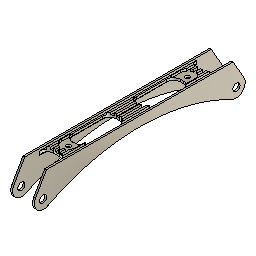
Sample Wall 270mm (Autodesk Fusion 360 archive; units mm, degrees)
design "Core-Large CDK"
Autodesk Fusion 360 part; units mm, degrees
sketch "Sketch1" plane through (0, 0, 0) normal (1, 0, 0) x (0, 1, 0)
  circle A0 centre (-135, -8) radius 5.05
  circle A1 centre (135, -8) radius 5.05
  arc A2 (128.3341, -19.5451) -> (-128.3341, -19.5451) centre (0, -267.4784) ccw
  line L0 (0, 25) -> (0, 11.7) construction
  arc A3 (-145.5683, -1.5) -> (-128.3341, -19.5451) centre (-134.31, -8) ccw
  line L1 (-20, 11.7) -> (20, 11.7) construction
  arc A4 (128.3341, -19.5451) -> (145.5683, -1.5) centre (134.31, -8) ccw
  line L2 (-135, -8) -> (135, -8) construction
  line L3 (-130.2685, 25) -> (130.2685, 25)
  line L4 (-132.0006, 22) -> (132.0006, 22)
  line L5 (-145.5683, -1.5) -> (-130.2685, 25)
  line L6 (145.5683, -1.5) -> (130.2685, 25)
  dimension "d3" = 10.1
  dimension "d4" = 135
  dimension "d5" = 10.1
  dimension "d6" = 135
  dimension "d146" = 13.3
  dimension "d154" = 13
  dimension "d155" = 25
  dimension "d156" = 33
  dimension "d157" = 120
  dimension "d158" = 13
  dimension "d159" = 120
  dimension "d160" = 0.69
  dimension "d161" = 0.69
  dimension "d162" = 3
  constraint horizontal L1
  constraint midpoint L0.end L1
  constraint tangent A2 A4
  constraint tangent A2 A3
  constraint coincident A0.centre L2.start
  constraint coincident A1.centre L2.end
  constraint horizontal L2
  constraint coincident L0.start L3
  constraint coincident L4.start L5
  constraint tangent A3 L5
  constraint coincident L4.end L6
  constraint tangent A4 L6
  constraint coincident A3.centre L2
  constraint coincident A4.centre L2
  constraint tangent A2 L1
  constraint horizontal L4
  measures "d3" diameter of A0
  measures "d4" horizontal distance of origin A0.centre
  measures "d5" diameter of A1
  measures "d6" horizontal distance of origin A1.centre
  measures "d146" distance of L0.start L0.end
  measures "d154" radius of A3
  measures "d155" distance of origin L0.start
  measures "d156" distance of L2 L3
  measures "d157" angle of L3 L5
  measures "d158" radius of A4
  measures "d159" angle of L3 L6
  measures "d160" distance of A3.centre A0.centre
  measures "d161" distance of A1.centre A4.centre
  measures "d162" distance of L3 L4
extrude "Extrude1" add sketch "Sketch1" along normal mid plane 33 makes body 1
sketch "Sketch3" plane through (0, 0, 0) normal (0, 1, 0) x (1, 0, 0)
  line L0 (-11.5, -19) -> (11.5, -19)
  line L1 (14, -16.5) -> (14, 23)
  line L2 (14, 23) -> (-14, 23)
  line L3 (-14, 23) -> (-14, -16.5)
  line L4 (-14, -19) -> (14, 23) construction
  line L5 (14, -19) -> (-14, 23) construction
  line L6 (-16.5, -22) -> (16.5, -22)
  line L7 (-11, -22) -> (-14, -22)
  line L8 (-14, -22) -> (-14, -25)
  line L9 (-14, -25) -> (-11, -25)
  line L10 (-11, -25) -> (-11, -22)
  line L11 (-11, -22) -> (-14, -25) construction
  line L12 (-14, -22) -> (-11, -25) construction
  line L13 (-16.5, 1.4544) -> (-16.5, -22)
  line L14 (14, -22) -> (11, -22)
  line L15 (11, -22) -> (11, -25)
  line L16 (11, -25) -> (14, -25)
  line L17 (14, -25) -> (14, -22)
  line L18 (14, -22) -> (11, -25) construction
  line L19 (11, -22) -> (14, -25) construction
  line L20 (16.5, -22) -> (16.5, 1.4544)
  arc A0 (-14, -16.5) -> (-11.5, -19) centre (-11.5, -16.5) ccw
  arc A1 (11.5, -19) -> (14, -16.5) centre (11.5, -16.5) ccw
  line L21 (5, -22) -> (8, -22)
  line L22 (8, -22) -> (8, -25)
  line L23 (8, -25) -> (5, -25)
  line L24 (5, -25) -> (5, -22)
  line L25 (5, -22) -> (8, -25) construction
  line L26 (8, -22) -> (5, -25) construction
  line L27 (-8, -22) -> (-5, -22)
  line L28 (-5, -22) -> (-5, -25)
  line L29 (-5, -25) -> (-8, -25)
  line L30 (-8, -25) -> (-8, -22)
  line L31 (-8, -22) -> (-5, -25) construction
  line L32 (-5, -22) -> (-8, -25) construction
  line L33 (-2, -22) -> (2, -22)
  line L34 (2, -22) -> (2, -25)
  line L35 (2, -25) -> (-2, -25)
  line L36 (-2, -25) -> (-2, -22)
  line L37 (-2, -22) -> (2, -25) construction
  line L38 (2, -22) -> (-2, -25) construction
  line L39 (-16.5, -25) -> (16.5, -25)
  point P0 (0, 2)
  point P1 (-12.5, -23.5)
  point P2 (12.5, -23.5)
  point P3 (0, -20.5)
  point P4 (6.5, -23.5)
  point P5 (-6.5, -23.5)
  point P6 (0, -23.5)
  dimension "d22" = 28
  dimension "d24" = 42
  dimension "d79" = 3
  dimension "d80" = 3
  dimension "d81" = 2.5
  dimension "d82" = 3
  dimension "d83" = 3
  dimension "d84" = 2.5
  dimension "d101" = 2.5
  dimension "d102" = 2.5
  dimension "d103" = 3
  dimension "d104" = 3
  dimension "d105" = 3
  dimension "d106" = 3
  dimension "d107" = 3
  dimension "d108" = 3
  dimension "d109" = 4
  dimension "d110" = 3
  dimension "d147" = 6
  constraint horizontal L0
  constraint perpendicular L0 L1
  constraint parallel L0 L2
  constraint parallel L1 L3
  constraint coincident L4 P0
  constraint coincident L5 P0
  constraint horizontal L7
  constraint perpendicular L7 L8
  constraint parallel L7 L9
  constraint parallel L8 L10
  constraint coincident L11 P1
  constraint coincident L12 P1
  constraint horizontal L14
  constraint perpendicular L14 L15
  constraint parallel L14 L16
  constraint parallel L15 L17
  constraint coincident L18 P2
  constraint coincident L19 P2
  constraint vertical origin P3
  constraint coincident L4.start L0
  constraint coincident L4.start L3
  constraint tangent L0 A0
  constraint tangent L3 A0
  constraint coincident L5.start L0
  constraint coincident L5.start L1
  constraint tangent L0 A1
  constraint tangent L1 A1
  constraint vertical origin P0
  constraint horizontal L21
  constraint perpendicular L21 L22
  constraint parallel L21 L23
  constraint parallel L22 L24
  constraint coincident L25 P4
  constraint coincident L26 P4
  constraint horizontal L27
  constraint perpendicular L27 L28
  constraint parallel L27 L29
  constraint parallel L28 L30
  constraint coincident L31 P5
  constraint coincident L32 P5
  constraint horizontal L33
  constraint perpendicular L33 L34
  constraint parallel L33 L35
  constraint parallel L34 L36
  constraint coincident L37 P6
  constraint coincident L38 P6
  constraint vertical P0 P6
  constraint horizontal L15.end L39.end
  constraint horizontal L34.end L39.end
  constraint horizontal L28.end L39.end
  measures "d22" distance of L1.end L2.end
  measures "d24" distance of L0 L2
  measures "d79" distance of L8.end L9.end
  measures "d80" distance of L7.end L8.end
  measures "d81" distance of L8 L13
  measures "d82" distance of L15.end L16.end
  measures "d83" distance of L14.end L15.end
  measures "d84" distance of L17 L20
  measures "d101" radius of A0
  measures "d102" radius of A1
  measures "d103" distance of L22.end L23.end
  measures "d104" distance of L21.end L22.end
  measures "d105" distance of L15 L22
  measures "d106" distance of L28.end L29.end
  measures "d107" distance of L27.end L28.end
  measures "d108" distance of L10 L30
  measures "d109" distance of L34.end L35.end
  measures "d110" distance of L33.end L34.end
  measures "d147" distance of L0 L39
extrude "Extrude2" cut sketch "Sketch3" along normal mid plane 360 contours L0 L1 L2 L3 A0 A1 | L6 L7 L8 L9 L10 L39 | L6 L27 L28 L29 L30 L39 | L6 L33 L34 L35 L36 L39 | L6 L21 L22 L23 L24 L39 | L6 L14 L15 L16 L17 L39 bodies 1
sketch "Sketch4" plane through (0, 0, 25) normal (0, 0, 1) x (-1, 0, 0)
  line L0 (-14, 122) -> (-16.5, 122)
  line L1 (-16.5, 122) -> (-16.5, -122)
  line L2 (-16.5, -122) -> (-14, -122)
  line L3 (16.5, -122) -> (16.5, 122)
  line L4 (0, 0) -> (0, -83.5) construction
  line L5 (0, 0) -> (0, 83.5) construction
  circle A0 centre (0, -83.5) radius 10.1
  circle A1 centre (0, -83.5) radius 3.1
  circle A2 centre (0, 83.5) radius 10.1
  circle A3 centre (0, 83.5) radius 3.1
  line L6 (-14, -122) -> (-14, 122)
  line L7 (14, 122) -> (14, -122)
  line L8 (14, -122) -> (16.5, -122)
  line L9 (16.5, 122) -> (14, 122)
  line L10 (-14, 25) -> (14, 25)
  line L11 (14, 25) -> (14, -25)
  line L12 (14, -25) -> (-14, -25)
  line L13 (-14, -25) -> (-14, 25)
  line L14 (-14, 25) -> (14, -25) construction
  line L15 (14, 25) -> (-14, -25) construction
  line L16 (-10.1, -63.49) -> (10.1, -63.49)
  line L17 (10.1, -63.49) -> (10.1, -83.5)
  line L18 (10.1, -83.5) -> (-10.1, -83.5)
  line L19 (-10.1, -83.5) -> (-10.1, -63.49)
  line L20 (-10.1, -63.49) -> (10.1, -83.5) construction
  line L21 (10.1, -63.49) -> (-10.1, -83.5) construction
  line L22 (-10.1, 83.5) -> (10.1, 83.5)
  line L23 (10.1, 83.5) -> (10.1, 63.48)
  line L24 (10.1, 63.48) -> (-10.1, 63.48)
  line L25 (-10.1, 63.48) -> (-10.1, 83.5)
  line L26 (-10.1, 83.5) -> (10.1, 63.48) construction
  line L27 (10.1, 83.5) -> (-10.1, 63.48) construction
  line L28 (-2, -132.0006) -> (2, -132.0006)
  line L29 (2, -132.0006) -> (2, 132.0006)
  line L30 (2, 132.0006) -> (-2, 132.0006)
  line L31 (-2, 132.0006) -> (-2, -132.0006)
  line L32 (-14, -130.2685) -> (-14, 130.2685)
  line L33 (-14, 130.2685) -> (-16.5, 130.2685)
  line L34 (-16.5, 130.2685) -> (-16.5, -130.2685)
  line L35 (-16.5, -130.2685) -> (-14, -130.2685)
  point P0 (0, -73.495)
  point P1 (0, 73.49)
  dimension "d28" = 83.5
  dimension "d29" = 83.5
  dimension "d30" = 20.2
  dimension "d31" = 6.2
  dimension "d32" = 20.2
  dimension "d33" = 6.2
  dimension "d97" = 28
  dimension "d98" = 50
  dimension "d125" = 20.01
  dimension "d126" = 20.2
  dimension "d127" = 20.2
  dimension "d128" = 20.02
  constraint coincident L4.start L5.start
  constraint vertical L4
  constraint parallel L4 L5
  constraint coincident L4.end A0.centre
  constraint concentric A0 A1
  constraint coincident L5.end A2.centre
  constraint concentric A2 A3
  constraint horizontal L10
  constraint perpendicular L10 L11
  constraint parallel L10 L12
  constraint parallel L11 L13
  constraint coincident L14 L4.start
  constraint coincident L15 L4.start
  constraint horizontal L16
  constraint perpendicular L16 L17
  constraint parallel L16 L18
  constraint parallel L17 L19
  constraint coincident L20 P0
  constraint coincident L21 P0
  constraint coincident L4 P0
  constraint horizontal L4.end L17.end
  constraint horizontal L22
  constraint perpendicular L22 L23
  constraint parallel L22 L24
  constraint parallel L23 L25
  constraint coincident L26 P1
  constraint coincident L27 P1
  constraint coincident L5 P1
  constraint horizontal L5.end L22.end
  measures "d28" distance of L4.start L4.end
  measures "d29" distance of L4.start L5.end
  measures "d30" diameter of A0
  measures "d31" diameter of A1
  measures "d32" diameter of A2
  measures "d33" diameter of A3
  measures "d97" distance of L11.end L12.end
  measures "d98" distance of L10.end L11.end
  measures "d125" distance of L16.end L17.end
  measures "d126" distance of L17 L19
  measures "d127" distance of L23.end L24.end
  measures "d128" distance of L22.end L23.end
extrude "Extrude3" cut sketch "Sketch4" against normal blind 100 contours A3 L22 L29 L31 | A3 L22 L31 | A1 L18 L31 | A1 L18 L29 L31 | A3 L22 L29 | A3 L22 L31 | A3 L22 L29 L31 | A1 L18 L29 | A1 L18 L31 | A1 L18 L29 L31 | A3 L22 L29 | A1 L18 L29 bodies 1
sketch "Sketch5" plane through (0, 0, 19) normal (0, 0, -1) x (1, 0, 0)
  circle A0 centre (0, -83.5) radius 3.1
  circle A1 centre (0, 83.5) radius 3.1
  circle A2 centre (0, -83.5) radius 13.1
  circle A3 centre (0, 83.5) radius 13.1
  line L0 (-11.5, 133.7326) -> (-11.5, -133.7326)
  line L1 (11.5, -133.7326) -> (11.5, 133.7326)
  line L2 (11.5, 133.7326) -> (-11.5, 133.7326)
  line L3 (-11.5, -133.7326) -> (11.5, -133.7326)
  dimension "d36" = 26.2
  dimension "d37" = 26.2
  constraint concentric A0 A2
  constraint concentric A1 A3
  measures "d36" diameter of A2
  measures "d37" diameter of A3
extrude "Extrude5" cut sketch "Sketch4" against normal blind 3 contours A2 L24 L29 L31 | A2 L24 L25 L31 | A0 L16 L19 L31 | A0 L16 L29 L31 | A2 L23 L24 L29 | A2 A3 L29 L31 | A2 A3 L22 L31 | A0 L16 L17 L29 | A0 A1 L18 L31 | A0 A1 L29 L31 | A2 A3 L22 L29 | A2 A3 L22 L31 | A0 A1 L18 L29 | A0 A1 L18 L31 | A2 A3 L22 L29 | A2 A3 L29 L31 | A0 A1 L18 L29 | A0 A1 L29 L31 bodies 1
sketch "Sketch6" plane through (0, 0, 25) normal (0, 0, 1) x (-1, 0, 0)
  line L0 (-14, 122) -> (-16.5, 122)
  line L1 (-16.5, 122) -> (-16.5, -122)
  line L2 (-16.5, -122) -> (-14, -122)
  line L3 (16.5, -122) -> (16.5, 122)
  line L4 (14, 149.5) -> (-14, 149.5)
  line L5 (-14, 149.5) -> (-14, 109.6)
  line L6 (-3.9, 99.5) -> (3.9, 99.5)
  line L7 (14, 109.6) -> (14, 149.5)
  line L8 (14, 149.5) -> (-14, 99.5) construction
  line L9 (-14, 149.5) -> (14, 99.5) construction
  arc A0 (3.9, 99.5) -> (14, 109.6) centre (3.9, 109.6) ccw
  arc A1 (-14, 109.6) -> (-3.9, 99.5) centre (-3.9, 109.6) ccw
  line L10 (14, -65.4) -> (14, -25.6)
  line L11 (-14, -25.6) -> (-14, -65.4)
  line L12 (-14, -149.5) -> (14, -149.5)
  line L13 (14, -149.5) -> (14, -109.6)
  line L14 (3.9, -99.5) -> (-3.9, -99.5)
  line L15 (-14, -109.6) -> (-14, -149.5)
  line L16 (-14, -149.5) -> (14, -99.5) construction
  line L17 (14, -149.5) -> (-14, -99.5) construction
  arc A2 (14, -109.6) -> (3.9, -99.5) centre (3.9, -109.6) ccw
  arc A3 (-3.9, -99.5) -> (-14, -109.6) centre (-3.9, -109.6) ccw
  line L18 (-14, -122) -> (-14, 122)
  line L19 (14, 122) -> (14, -122)
  line L20 (14, -122) -> (16.5, -122)
  line L21 (16.5, 122) -> (14, 122)
  line L22 (-1.9, 75.5) -> (1.9, 75.5)
  line L23 (12, 65.4) -> (12, 24.1)
  line L24 (1.9, 14) -> (-1.9, 14)
  line L25 (-12, 24.1) -> (-12, 65.4)
  line L26 (-12, 75.5) -> (12, 14) construction
  line L27 (12, 75.5) -> (-12, 14) construction
  arc A4 (1.9, 14) -> (12, 24.1) centre (1.9, 24.1) ccw
  arc A5 (-12, 24.1) -> (-1.9, 14) centre (-1.9, 24.1) ccw
  arc A6 (-1.9, 75.5) -> (-12, 65.4) centre (-1.9, 65.4) ccw
  arc A7 (12, 65.4) -> (1.9, 75.5) centre (1.9, 65.4) ccw
  line L28 (-1.9, -14) -> (1.9, -14)
  line L29 (12, -24.1) -> (12, -65.4)
  line L30 (1.9, -75.5) -> (-1.9, -75.5)
  line L31 (-12, -65.4) -> (-12, -24.1)
  line L32 (-12, -14) -> (12, -75.5) construction
  line L33 (12, -14) -> (-12, -75.5) construction
  arc A8 (1.9, -75.5) -> (12, -65.4) centre (1.9, -65.4) ccw
  arc A9 (-12, -65.4) -> (-1.9, -75.5) centre (-1.9, -65.4) ccw
  arc A10 (-1.9, -14) -> (-12, -24.1) centre (-1.9, -24.1) ccw
  arc A11 (12, -24.1) -> (1.9, -14) centre (1.9, -24.1) ccw
  line L34 (-14, -130.2685) -> (-14, 130.2685)
  line L35 (-14, 130.2685) -> (-16.5, 130.2685)
  line L36 (-16.5, 130.2685) -> (-16.5, -130.2685)
  line L37 (-16.5, -130.2685) -> (-14, -130.2685)
  point P0 (0, 45.5)
  point P1 (0, 124.5)
  point P2 (0, -124.5)
  point P3 (0, 83.5)
  point P4 (0, -83.5)
  point P5 (0, 44.75)
  point P6 (0, -44.75)
  dimension "d53" = 28
  dimension "d54" = 50
  dimension "d56" = 10.1
  dimension "d57" = 10.1
  dimension "d65" = 28
  dimension "d66" = 50
  dimension "d68" = 10.1
  dimension "d69" = 10.1
  dimension "d91" = 16
  dimension "d94" = 16
  dimension "d131" = 24
  dimension "d132" = 10.1
  dimension "d133" = 10.1
  dimension "d134" = 8
  dimension "d135" = 14
  dimension "d136" = 24
  dimension "d137" = 14
  dimension "d138" = 8
  dimension "d139" = 10.1
  constraint vertical origin P0
  constraint horizontal L4
  constraint perpendicular L4 L5
  constraint parallel L4 L6
  constraint parallel L5 L7
  constraint coincident L8 P1
  constraint coincident L9 P1
  constraint coincident L9.end L7
  constraint coincident L9.end L6
  constraint tangent L7 A0
  constraint tangent L6 A0
  constraint coincident L8.end L5
  constraint coincident L8.end L6
  constraint tangent L5 A1
  constraint tangent L6 A1
  constraint parallel L10 L11
  constraint horizontal L12
  constraint perpendicular L12 L13
  constraint parallel L12 L14
  constraint parallel L13 L15
  constraint coincident L16 P2
  constraint coincident L17 P2
  constraint coincident L16.end L13
  constraint coincident L16.end L14
  constraint tangent L13 A2
  constraint tangent L14 A2
  constraint coincident L17.end L14
  constraint coincident L17.end L15
  constraint tangent L14 A3
  constraint tangent L15 A3
  constraint vertical P1 P3
  constraint vertical P2 P4
  constraint horizontal L22
  constraint perpendicular L22 L23
  constraint parallel L22 L24
  constraint parallel L23 L25
  constraint coincident L26 P5
  constraint coincident L27 P5
  constraint coincident L26.end L24
  constraint coincident L26.end L23
  constraint tangent L24 A4
  constraint tangent L23 A4
  constraint coincident L27.end L24
  constraint coincident L27.end L25
  constraint tangent L24 A5
  constraint tangent L25 A5
  constraint coincident L26.start L25
  constraint coincident L26.start L22
  constraint tangent L25 A6
  constraint tangent L22 A6
  constraint equal A5 A6
  constraint coincident L27.start L22
  constraint coincident L27.start L23
  constraint tangent L22 A7
  constraint tangent L23 A7
  constraint equal A5 A7
  constraint vertical P3 P5
  constraint horizontal L28
  constraint perpendicular L28 L29
  constraint parallel L28 L30
  constraint parallel L29 L31
  constraint coincident L32 P6
  constraint coincident L33 P6
  constraint coincident L32.end L30
  constraint coincident L32.end L29
  constraint tangent L30 A8
  constraint tangent L29 A8
  constraint coincident L33.end L30
  constraint coincident L33.end L31
  constraint tangent L30 A9
  constraint tangent L31 A9
  constraint equal A8 A9
  constraint coincident L32.start L31
  constraint coincident L32.start L28
  constraint tangent L31 A10
  constraint tangent L28 A10
  constraint equal A8 A10
  constraint coincident L33.start L29
  constraint coincident L33.start L28
  constraint tangent L29 A11
  constraint tangent L28 A11
  constraint equal A8 A11
  constraint vertical P4 P6
  measures "d53" distance of L8.end L9.end
  measures "d54" distance of L4.end L8.end
  measures "d56" radius of A0
  measures "d57" radius of A1
  measures "d65" distance of L16.end L17.end
  measures "d66" distance of L12.end L16.end
  measures "d68" radius of A2
  measures "d69" radius of A3
  measures "d91" distance of L6 P3
  measures "d94" distance of L14 P4
  measures "d131" distance of L26.end L27.end
  measures "d132" radius of A4
  measures "d133" radius of A5
  measures "d134" distance of P3 L22
  measures "d135" distance of origin L24
  measures "d136" distance of L32.end L33.end
  measures "d137" distance of origin L28
  measures "d138" distance of P4 L30
  measures "d139" radius of A8
extrude "Extrude6" cut sketch "Sketch6" against normal blind 110 contours L4 L5 L6 L7 A0 A1 L18 L19 L34 | L12 L13 L14 L15 A2 A3 L18 L19 L34 | L22 L23 L24 L25 A4 A5 A6 A7 | L28 L29 L30 L31 A8 A9 A10 A11 bodies 1
sketch "Sketch7" plane through (0, 0, 0) normal (1, 0, 0) x (0, 1, 0)
  circle A0 centre (-135, -8) radius 32.5
  circle A1 centre (135, -8) radius 36
  circle A2 centre (-55, -8) radius 32.5
  circle A3 centre (55, -8) radius 32.5
  point P0 (-135, -8)
  point P1 (135, -8)
  dimension "d72" = 65
  dimension "d73" = 72
  dimension "d140" = 65
  dimension "d141" = 80
  dimension "d142" = 65
  dimension "d143" = 80
  constraint coincident P0 A0.centre
  constraint coincident P1 A1.centre
  constraint horizontal P0 A2.centre
  constraint horizontal P1 A3.centre
  measures "d72" diameter of A0
  measures "d73" diameter of A1
  measures "d140" diameter of A2
  measures "d141" distance of P0 A2.centre
  measures "d142" diameter of A3
  measures "d143" distance of P1 A3.centre
extrude "Extrude1'" add sketch "Sketch7" along normal mid plane 24 separate body makes body 2 at (12, -141.3222, -15.3685) makes body 3 at (12, 144.7808, -3.0287) makes body 4 at (12, -63.3736, 0.4698) makes body 5 at (12, 63.2133, 1.1724) in component "Wheels"
fillet "Fillet1" radius 6 8 edges at (12, -165.3006, -19.7525) (-12, -165.3006, 3.7525) (-12, 101.4362, 5.0182) (12, 101.4362, -21.0182) (-12, -85.3006, 3.7525) (12, -85.3006, -19.7525) (12, 24.6994, -19.7525) (-12, 24.6994, 3.7525) on bodies 2 3 4 5 in component "Wheels"
component "Wheels" placed x (1, 0, 0) y (0, 1, 0) z (0, 0, 1) at (0, 0, 0)
named bodies: "Core-Large"
